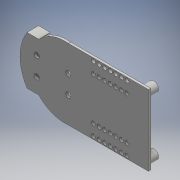
# Autodesk Inventor part: baseChassis322016
Saved by Autodesk Inventor 2016 (Build 200138000, 138)
## iProperties
Created: 2016-03-02
Part Number: baseChassis322016
Material: Generic
Document SubType Name: Modeling
Designer: mkepler
Density: 1 g/cm^3
Appearance: Default
Author: mkepler
Autodesk Inventor part; units mm, degrees
ref_plane "YZ Plane" through (0, 0, 0) normal (1, 0, 0) x (0, 1, 0)
ref_plane "XZ Plane" through (0, 0, 0) normal (0, 1, 0) x (-1, 0, 0)
ref_plane "XY Plane" through (0, 0, 0) normal (0, 0, 1) x (1, 0, 0)
sketch "Sketch1" plane through (0, 0, 0) normal (0, 1, 0) x (-1, 0, 0)
  line L0 (0, 0) -> (86, 0)
  line L1 (0, 0) -> (0, -76)
  line L2 (86, -76) -> (0, -76)
  arc A0 (86, -76) -> (86, 0) centre (89.8131, -38) ccw
  line L3 (86, -76) -> (86, -86)
  line L4 (86, 0) -> (86, 10)
  arc A1 (130.3413, -64) -> (130.3413, -12) centre (89.8131, -38) ccw
  line L5 (86, 0) -> (86, -12)
  line L6 (86, -76) -> (86, -64)
  line L7 (117.787, -12) -> (130.3413, -12)
  line L8 (117.787, -64) -> (130.3413, -64)
  line L9 (117.787, -12) -> (130.3413, -12)
  line L10 (117.787, -64) -> (130.3413, -64)
  line L11 (130.3413, -12) -> (117.787, -12)
  line L12 (130.3413, -64) -> (117.787, -64)
  arc A2 (117.787, -64) -> (117.787, -12) centre (89.8131, -38) ccw
  arc A3 (130.3413, -64) -> (130.3413, -12) centre (89.8131, -38) ccw
  dimension "d1" = 86
  dimension "d2" = 76
  dimension "d3" = 10
  dimension "d4" = 10
  dimension "d6" = 12
  dimension "d7" = 12
  constraints: 26 end point, 12 point on circle, 5 vertical, 4 centre point, 3 equal length, 3 horizontal, 2 concentric, 1 perpendicular
  measures "d1" distance of L0.start L0.end
  measures "d2" distance of L0.start L1.end
  measures "d3" distance of L2.start L3.end
  measures "d4" distance of L0.end L4.end
  measures "d6" distance of L0.end L5.end
  measures "d7" distance of L2.start L6.end
extrude "Extrusion1" add sketch "Sketch1" along normal blind 2.4
sketch "Sketch2" plane through (0, 2.4, 0) normal (0, 1, 0) x (1, 0, 0)
  circle A0 centre (-6.5, 6.5) radius 5
  circle A1 centre (-6.5, 69.5) radius 5
  line L0 (-86, 0) -> (0, 0) projected
  line L1 (0, 0) -> (0, 76) projected
  arc A2 (-117.787, 64) -> (-117.787, 12) centre (-89.7207, 38) ccw
  line L2 (-130.3413, 12) -> (-117.787, 12) projected
  line L3 (-130.3413, 12) -> (-117.787, 12)
  line L4 (-117.787, 64) -> (-130.3413, 64) projected
  line L5 (-130.3413, 64) -> (-117.787, 64)
  arc A3 (-130.3413, 64) -> (-130.3413, 12) centre (-89.8131, 38) ccw
  dimension "d10" = 10
  dimension "d11" = 10
  dimension "d12" = 63
  dimension "d13" = 6.5
  dimension "d14" = 6.5
  dimension "d15" = 6.5
  constraints: 4 centre point, 4 end point, 4 point on circle, 2 horizontal
  measures "d10" diameter of A0
  measures "d11" diameter of A1
  measures "d12" distance of A1.centre A0.centre
  measures "d13" distance from line of L0 A0.centre
  measures "d14" distance from line of L1 A0.centre
  measures "d15" distance from line of L1 A1.centre
extrude "Extrusion2" add sketch "Sketch2" along normal blind 10
sketch "Sketch4" plane through (-6.5, 12.4, -6.5) normal (0, 1, 0) x (1, 0, 0)
  circle A0 centre (0, 0) radius 3.25
  circle A1 centre (0, 63) radius 5 projected
  circle A2 centre (0, 63) radius 3.25
  line L0 (0, 0) -> (0, 63)
  line L1 (6.5, -6.5) -> (6.5, 69.5) projected
  line L2 (0, 31.5) -> (-127.167, 31.5)
  circle A3 centre (-127.167, 31.5) radius 3.25
  dimension "d20" = 6.5
  dimension "d21" = 6.5
  dimension "d22" = 127.167
  dimension "d23" = 6.5
  dimension "d70" = 63
  constraints: 4 end point, 3 centre point, 2 coincident, 1 horizontal, 1 midpoint, 1 parallel
  measures "d20" diameter of A0
  measures "d21" diameter of A2
  measures "d22" distance of L2.start L2.end
  measures "d23" diameter of A3
  measures "d70" distance of A2.centre L0.start
hole "Hole1" at (-133.667, 12.4, -38) at (-6.5, 12.4, -69.5) at (-6.5, 12.4, -6.5) direction (0, -1, 0) diameter 6.5 depth 9
sketch "Sketch5" plane through (0, 2.4, 0) normal (0, 1, 0) x (1, 0, 0)
  line L0 (-86, 0) -> (0, 0) projected
  line L1 (-55.3616, 0) -> (-55.3616, 76)
  line L2 (0, 76) -> (-86, 76) projected
  line L3 (-55.3616, 38) -> (-127.9792, 38)
  arc A0 (-117.787, 64) -> (-117.787, 12) centre (-89.7207, 38) ccw projected
  arc A1 (-117.787, 64) -> (-117.787, 12) centre (-89.7207, 38) ccw projected
  arc A2 (-117.787, 12) -> (-86, 0) centre (-89.8131, 38) ccw projected
  line L4 (-86, 0) -> (0, 0) projected
  line L5 (0, 0) -> (0, 76) projected
  line L6 (0, 76) -> (-86, 76) projected
  arc A3 (-86, 76) -> (-117.787, 64) centre (-89.8131, 38) ccw projected
  circle A4 centre (-6.5, 69.5) radius 5 projected
  circle A5 centre (-6.5, 6.5) radius 5 projected
  circle A6 centre (-119.9244, 28) radius 2.75
  line L7 (-119.9244, 28) -> (-119.9244, 38)
  circle A7 centre (-119.9244, 48) radius 2.75
  circle A8 centre (-85.9244, 28) radius 2.75
  circle A9 centre (-85.9244, 48) radius 2.75
  dimension "d36" = 5.5
  dimension "d38" = 5.5
  dimension "d39" = 10
  dimension "d40" = 10
  dimension "d41" = 5.5
  dimension "d42" = 5.5
  dimension "d43" = 34
  dimension "d44" = 34
  constraints: 6 end point, 4 centre point, 3 point on line, 2 perpendicular, 1 midpoint, 1 point on circle, 1 vertical
  measures "d36" diameter of A6
  measures "d38" diameter of A7
  measures "d39" distance of L7.end A7.centre
  measures "d40" distance of L7.end L7.start
  measures "d41" diameter of A8
  measures "d42" diameter of A9
  measures "d43" distance of A8.centre L7.start
  measures "d44" distance of A9.centre A7.centre
hole "Hole2" at (-119.9244, 2.4, -28) at (-119.9244, 2.4, -48) at (-85.9244, 2.4, -48) at (-85.9244, 2.4, -28) direction (0, -1, 0) diameter 5.5 end through all
sketch "Sketch6" plane through (0, 2.4, 0) normal (0, 1, 0) x (1, 0, 0)
  line L0 (-16.1203, 0) -> (-16.1203, 27)
  circle A0 centre (-23, 61) radius 2.2
  line L1 (0, 0) -> (0, 76) projected
  line L2 (0, 76) -> (-86, 76) projected
  circle A1 centre (-35, 61) radius 2.2
  circle A2 centre (-47, 61) radius 2.2
  circle A3 centre (-59, 61) radius 2.2
  line L3 (0, 0) -> (0, 76) projected
  line L4 (0, 38) -> (-47, 38)
  circle A4 centre (-23, 15) radius 2.2
  circle A5 centre (-35, 15) radius 2.2
  circle A6 centre (-47, 15) radius 2.2
  circle A7 centre (-59, 15) radius 2.2
  line L5 (-47, 38) -> (-86, 38)
  line L6 (-35, 61) -> (-35, 73)
  circle A8 centre (-35, 73) radius 2.2
  circle A9 centre (-47, 73) radius 2.2
  circle A10 centre (-35, 3) radius 2.2
  circle A11 centre (-47, 3) radius 2.2
  circle A12 centre (-53, 61) radius 2.2
  circle A13 centre (-41, 61) radius 2.2
  circle A14 centre (-29, 61) radius 2.2
  line L7 (-47, 61) -> (-47, 73)
  line L8 (-47, 67) -> (-37.2, 67)
  circle A15 centre (-23, 73) radius 2.2
  circle A16 centre (-35, 73) radius 2.2
  circle A17 centre (-47, 73) radius 2.2
  circle A18 centre (-59, 73) radius 2.2
  line L9 (-35, 73) -> (-35, 61)
  circle A19 centre (-53, 73) radius 2.2
  circle A20 centre (-41, 73) radius 2.2
  circle A21 centre (-29, 73) radius 2.2
  circle A22 centre (-23, 15) radius 2.2
  circle A23 centre (-35, 15) radius 2.2
  circle A24 centre (-47, 15) radius 2.2
  circle A25 centre (-59, 15) radius 2.2
  circle A26 centre (-35, 3) radius 2.2
  circle A27 centre (-53, 15) radius 2.2
  circle A28 centre (-41, 15) radius 2.2
  circle A29 centre (-29, 15) radius 2.2
  circle A30 centre (-59, 3) radius 2.2
  circle A31 centre (-53, 3) radius 2.2
  circle A32 centre (-47, 3) radius 2.2
  circle A33 centre (-41, 3) radius 2.2
  circle A34 centre (-29, 3) radius 2.2
  circle A35 centre (-23, 3) radius 2.2
  dimension "d52" = 27
  dimension "d54" = 4.4
  dimension "d57" = 4.4
  dimension "d59" = 4.4
  dimension "d61" = 4.4
  dimension "d71" = 23
  dimension "d73" = 23
  dimension "d74" = 23
  dimension "d75" = 23
  dimension "d76" = 12
  dimension "d77" = 4.4
  dimension "d78" = 4.4
  dimension "d79" = 4.4
  dimension "d80" = 6
  dimension "d81" = 4.4
  dimension "d82" = 6
  dimension "d83" = 4.4
  dimension "d84" = 6
  constraints: 36 centre point, 29 symmetric about line, 14 end point, 3 coincident, 3 horizontal, 2 midpoint, 2 vertical, 1 perpendicular, 27 other
  measures "d52" distance of L0.start L0.end
  measures "d54" diameter of A0
  measures "d57" diameter of A1
  measures "d59" diameter of A2
  measures "d61" diameter of A3
  measures "d71" distance from line of L4 A3.centre
  measures "d73" distance of L4.end L7.start
  measures "d74" distance from line of L4 L6.start
  measures "d75" distance from line of L4 A0.centre
  measures "d76" distance of L6.start L6.end
  measures "d77" diameter of A8
  measures "d78" diameter of A9
  measures "d79" diameter of A12
  measures "d80" distance of A12.centre A3.centre
  measures "d81" diameter of A13
  measures "d82" distance of A13.centre L7.start
  measures "d83" diameter of A14
  measures "d84" distance of L6.start A14.centre
hole "Hole3" at (-59, 2.4, -15) at (-47, 2.4, -15) at (-35, 2.4, -15) at (-23, 2.4, -15) at (-23, 2.4, -61) at (-35, 2.4, -61) at (-47, 2.4, -61) at (-59, 2.4, -61) at (-47, 2.4, -3) at (-35, 2.4, -3) at (-35, 2.4, -73) at (-47, 2.4, -73) at (-59, 2.4, -3) at (-53, 2.4, -3) at (-53, 2.4, -15) at (-41, 2.4, -15) at (-41, 2.4, -3) at (-29, 2.4, -3) at (-23, 2.4, -3) at (-29, 2.4, -15) at (-59, 2.4, -73) at (-53, 2.4, -73) at (-53, 2.4, -61) at (-41, 2.4, -61) at (-41, 2.4, -73) at (-29, 2.4, -73) at (-29, 2.4, -61) at (-23, 2.4, -73) direction (0, -1, 0) diameter 4.4 end through all
body "Solid1"
